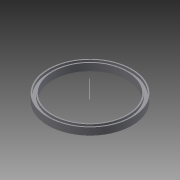
# Autodesk Inventor part: Cap
Saved by Autodesk Inventor 2015 (Build 190159000, 159)
## iProperties
Created: 2014-07-08
Part Number: Cap
Material: Generic
Document SubType Name: Modeling
Designer: I Rabey
Density: 1 g/cm^3
Appearance: Default
Author: I Rabey
Autodesk Inventor part; units mm, degrees
ref_plane "YZ Plane" through (0, 0, 0) normal (1, 0, 0) x (0, 1, 0)
ref_plane "XY Plane" through (0, 0, 0) normal (0, 0, 1) x (1, 0, 0)
sketch "Sketch14" plane through (0, 0, 0) normal (0, 1, 0) x (-1, 0, 0)
  circle A0 centre (0, 0) radius 26
  circle A1 centre (0, 0) radius 29.5
  dimension "d122" = 52
  dimension "d123" = 59
  constraints: 2 centre point, 2 coincident
  measures "d122" diameter of A0
  measures "d123" diameter of A1
extrude "Extrusion3" add sketch "Sketch14" along normal blind 5
sketch "Sketch15" plane through (0, 5, 0) normal (0, 1, 0) x (1, 0, 0)
  circle A0 centre (0, 0) radius 26.85
  circle A1 centre (0, 0) radius 28.65
  dimension "d126" = 53.7
  dimension "d127" = 57.3
  constraints: 2 centre point, 2 coincident
  measures "d126" diameter of A0
  measures "d127" diameter of A1
extrude "Extrusion4" cut sketch "Sketch15" against normal blind 1.8
ref_plane "Work Plane1" through (0, 4.1, 0) normal (0, 1, 0) x (-1, 0, 0)
sketch "Sketch16" plane through (0, 0, 0) normal (0, -1, 0) x (1, 0, 0)
  circle A0 centre (28, 0) radius 1
  point P0 (0, 0)
  dimension "d131" = 2
  dimension "d132" = 28
  constraints: 1 centre point
  measures "d131" diameter of A0
  measures "d132" distance of point (0, 0) A0.centre
hole "Hole12" at (28, 0, 0) direction (0, 1, 0) diameter 2 depth 2
sketch "Sketch17" plane through (0, 0, 0) normal (0, -1, 0) x (1, 0, 0)
  circle A0 centre (0, -28) radius 1
  point P0 (0, 0)
  dimension "d140" = 2
  dimension "d141" = 28
  constraints: 1 centre point
  measures "d140" diameter of A0
  measures "d141" distance of A0.centre point (0, 0)
hole "Hole13" at (0, 0, -28) direction (0, 1, 0) diameter 2 depth 2
sketch "Sketch18" plane through (0, 0, 0) normal (0, -1, 0) x (1, 0, 0)
  circle A0 centre (0, 28) radius 1
  point P0 (0, 0)
  dimension "d149" = 2
  dimension "d150" = 28
  constraints: 1 centre point
  measures "d149" diameter of A0
  measures "d150" distance of point (0, 0) A0.centre
hole "Hole14" at (0, 0, 28) direction (0, 1, 0) diameter 2 depth 2
sketch "Sketch19" plane through (0, 0, 0) normal (0, -1, 0) x (1, 0, 0)
  circle A0 centre (-28, 0) radius 1
  point P0 (0, 0)
  dimension "d158" = 2
  dimension "d159" = 28
  constraints: 1 centre point
  measures "d158" diameter of A0
  measures "d159" distance of point (0, 0) A0.centre
hole "Hole15" at (-28, 0, 0) direction (0, 1, 0) diameter 2 depth 2
thread "Thread5" size "M2x0.4" class "6H" standard "ANSI Metric M Profile" full length
thread "Thread6" size "M2x0.4" class "6H" standard "ANSI Metric M Profile" full length
thread "Thread7" size "M2x0.4" class "6H" standard "ANSI Metric M Profile" full length
thread "Thread8" size "M2x0.4" class "6H" standard "ANSI Metric M Profile" full length
body "Solid3"
